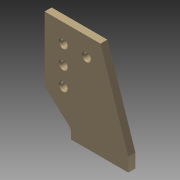
# Autodesk Inventor part: Uprights
Saved by Autodesk Inventor 2012 (Build 160160000, 160)
## iProperties
Created: 2013-05-09
Part Number: Uprights
Material: Default
Document SubType Name: Modeling
Designer: Fabian
Density: 1 g/cm^3
Author: Fabian
Autodesk Inventor part; units mm, degrees
ref_plane "YZ Plane" through (0, 0, 0) normal (1, 0, 0) x (0, 1, 0)
ref_plane "XZ Plane" through (0, 0, 0) normal (0, 1, 0) x (-1, 0, 0)
ref_plane "XY Plane" through (0, 0, 0) normal (0, 0, 1) x (1, 0, 0)
sketch "Sketch1" plane through (0, 0, 0) normal (0, 0, 1) x (1, 0, 0)
  line L0 (-50.4258, 38.8802) -> (105.7842, 38.8802)
  line L1 (105.7842, 38.8802) -> (105.7842, 0.7802)
  line L2 (105.7842, 0.7802) -> (-50.4258, 0.7802)
  line L3 (-50.4258, 0.7802) -> (-50.4258, 38.8802)
  line L4 (-122.8158, 267.4802) -> (29.5842, 267.4802)
  line L5 (29.5842, 267.4802) -> (29.5842, 165.8802)
  line L6 (29.5842, 165.8802) -> (-122.8158, 165.8802)
  line L7 (-122.8158, 165.8802) -> (-122.8158, 267.4802)
  line L8 (29.5842, 267.4802) -> (105.7842, 38.8802)
  line L9 (-122.8158, 165.8802) -> (-50.4258, 102.3802)
  line L10 (-50.4258, 102.3802) -> (-50.4258, 38.8802)
  point P0 (0, 0)
  dimension "d0" = 156.21
  dimension "d1" = 38.1
  dimension "d2" = 101.6
  dimension "d3" = 152.4
  dimension "d4" = 228.6
  dimension "d5" = 76.2
  dimension "d19" = 63.5
  constraints: 22 end point, 4 parallel, 2 horizontal, 2 perpendicular, 1 collinear
  measures "d0" distance of L0.start L0.end
  measures "d1" distance of L2.end L0.start
  measures "d2" distance of L4.end L5.end
  measures "d3" distance of L4.start L4.end
  measures "d4" distance between parallel lines of L0 L4
  measures "d5" distance between parallel lines of L1 L5
  measures "d19" distance of L9.end L0.start
extrude "Extrusion1" add sketch "Sketch1" along normal blind 19.05
sketch "Sketch5" plane through (0, 0, 0) normal (0, 0, -1) x (-1, 0, 0)
  line L0 (50.4258, 102.3802) -> (50.4258, 0.7802) projected
  line L1 (122.8158, 165.8802) -> (50.4258, 102.3802) projected
  line L2 (122.8158, 165.8802) -> (122.8158, 89.6802)
  line L3 (122.8158, 89.6802) -> (50.4258, 26.1802)
  point P0 (0, 0)
  dimension "d40" = 76.2
  dimension "d41" = 76.2
  constraints: 4 end point, 1 parallel, 1 point on line
  measures "d40" distance of L1.start L2.end
  measures "d41" distance of L3.end L0.start
extrude "Extrusion3" add sketch "Sketch5" against normal blind 19.05
sketch "Sketch6" plane through (0, 0, 19.05) normal (0, 0, 1) x (1, 0, 0)
  line L0 (-122.8158, 267.4802) -> (29.5842, 267.4802) projected
  line L1 (-122.8158, 89.6802) -> (-122.8158, 267.4802) projected
  point P0 (0, 0)
  point P1 (-72.0158, 216.6802)
  point P2 (-8.5158, 216.6802)
  point P3 (-72.0158, 115.0802)
  point P4 (-72.0158, 165.8802)
  dimension "d44" = 50.8
  dimension "d45" = 50.8
  dimension "d46" = 50.8
  dimension "d47" = 50.8
  dimension "d48" = 50.8
  dimension "d49" = 50.8
  dimension "d50" = 50.8
  dimension "d51" = 63.5
  measures "d44" distance from line of L0 point (-72.016, 216.68)
  measures "d45" distance from line of L0 point (-8.516, 216.68)
  measures "d46" distance from line of L1 point (-72.016, 216.68)
  measures "d47" distance from line of L1 point (-72.016, 165.88)
  measures "d48" distance from line of L1 point (-72.016, 115.08)
  measures "d49" distance of point (-72.016, 165.88) point (-72.016, 216.68)
  measures "d50" distance of point (-72.016, 115.08) point (-72.016, 165.88)
  measures "d51" distance of point (-72.016, 216.68) point (-8.516, 216.68)
hole "Hole3" at (-72.0158, 216.6802, 19.05) at (-8.5158, 216.6802, 19.05) at (-72.0158, 115.0802, 19.05) at (-72.0158, 165.8802, 19.05) direction (0, 0, -1) diameter 19.05 end through all
fillet "Fillet1" radius 25.4 1 edges at (-50.4258, 26.1802, 9.525)
chamfer "Chamfer1" distance 2.54 angle 45 8 edges at (-8.5158, 226.2052, 0) (-72.0158, 226.2052, 0) (-72.0158, 175.4052, 0) (-72.0158, 124.6052, 0) (-72.0158, 226.2052, 19.05) (-8.5158, 226.2052, 19.05) (-72.0158, 175.4052, 19.05) (-72.0158, 124.6052, 19.05)
equation "\"d45\" = d44"
equation "\"d46\" = d44"
equation "\"d47\" = d44"
equation "\"d48\" = d44"
body "Solid1"
